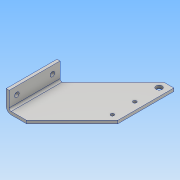
# Autodesk Inventor part: Pancake_Bracket
Saved by Autodesk Inventor 2018.1 (Build 221171000, 171)
## iProperties
Created: 2019-02-27
Part Number: Pancake_Bracket
Material: Aluminum 6061
Document SubType Name: Modeling
Designer: James
Density: 2.7 g/cm^3
Appearance: Aluminum - Flat
Author: James
Autodesk Inventor part; units mm, degrees
ref_plane "YZ Plane" through (0, 0, 0) normal (1, 0, 0) x (0, 1, 0)
ref_plane "XZ Plane" through (0, 0, 0) normal (0, 1, 0) x (-1, 0, 0)
ref_plane "XY Plane" through (0, 0, 0) normal (0, 0, 1) x (1, 0, 0)
sketch "Sketch1" plane through (0, 0, 0) normal (0, 0, 1) x (1, 0, 0)
  line L0 (0, 0) -> (65, 0)
  line L1 (65, 0) -> (65, 100)
  line L2 (65, 100) -> (0, 100)
  line L3 (0, 100) -> (0, 0)
  line L4 (0, 50) -> (5, 50)
  line L5 (5, 50) -> (55, 100)
  dimension "d0" = 65
  dimension "d1" = 100
  dimension "d28" = 45
  dimension "d29" = 50
  dimension "d30" = 5
  constraints: 12 end point, 2 horizontal, 2 parallel, 1 midpoint, 1 perpendicular, 1 point on line
  measures "d0" distance of L1.end L2.end
  measures "d1" distance of L0.end L1.end
  measures "d28" angle of L5 L2
  measures "d29" distance between parallel lines of L0 L4
  measures "d30" distance of L4.start L4.end
extrude "Extrusion1" add sketch "Sketch1" along normal blind 3 contours L3 L4 L5 L2 L1 L0
sketch "Sketch2" plane through (0, 0, 3) normal (0, 0, 1) x (1, 0, 0)
  line L0 (0, 0) -> (65, 0) projected
  line L1 (0, 0) -> (3, 0)
  line L2 (3, 0) -> (3, 50)
  line L3 (3, 50) -> (0, 50)
  line L4 (0, 50) -> (0, 0)
  dimension "d4" = 3
  dimension "d5" = 50
  constraints: 8 end point, 2 parallel, 1 horizontal, 1 perpendicular
  measures "d4" distance of L2.end L3.end
  measures "d5" distance of L1.end L2.end
extrude "Extrusion2" add sketch "Sketch2" along normal blind 17
chamfer "Chamfer2" distance 45 angle 45 1 edges at (65, 0, 1.5)
sketch "Sketch4" plane through (3, 0, 3) normal (1, 0, 0) x (0, 0, -1)
  line L0 (-17, 0) -> (-17, 50) projected
  line L1 (0, 50) -> (-17, 50) projected
  line L2 (0, 0) -> (-17, 0) projected
  point P0 (3, 0)
  point P1 (-9.5, 42.5)
  point P2 (-9.5, 7.5)
  dimension "d31" = 7.5
  dimension "d32" = 7.5
  dimension "d33" = 7.5
  dimension "d34" = 35
  constraints: 1 vertical alignment
  measures "d31" distance from line of L0 point (-9.5, 42.5)
  measures "d32" distance from line of point (-9.5, 42.5) L1
  measures "d33" distance from line of L2 point (-9.5, 7.5)
  measures "d34" distance of point (-9.5, 42.5) point (-9.5, 7.5)
hole "Hole1" at (3, 42.5, 12.5) at (3, 7.5, 12.5) direction (-1, 0, 0) diameter 4.5 end through all clearance for "Flat Head Machine Screw" size "M4" standard "Ansi Metric M Profile"
sketch "Sketch3" plane through (0, 0, 3) normal (0, 0, 1) x (1, 0, 0)
  line L0 (3, 0) -> (3, 50) projected
  line L1 (0, 50) -> (0, 0) projected
  line L2 (3, 50) -> (0, 50) projected
  point P0 (57.5, 93)
  dimension "d10" = 57.5
  dimension "d42" = 43
  measures "d10" distance from line of point (57.5, 93) L1
  measures "d42" distance from line of L2 point (57.5, 93)
hole "Hole2" at (57.5, 93, 3) direction (0, 0, -1) diameter 6 end through all
sketch "Sketch5" plane through (0, 0, 3) normal (0, 0, 1) x (1, 0, 0)
  circle A0 centre (57.5, 93) radius 3 projected
  point P0 (0, 0)
  point P1 (57.5, 69)
  point P2 (57.5, 47)
  dimension "d50" = 24
  dimension "d51" = 22
  constraints: 2 vertical alignment
  measures "d50" distance of point (57.5, 69) A0.centre
  measures "d51" distance of point (57.5, 47) point (57.5, 69)
hole "Hole3" at (57.5, 69, 3) at (57.5, 47, 3) direction (0, 0, -1) diameter 3.4 end through all clearance for "Flat Head Machine Screw" size "M3" standard "Ansi Metric M Profile"
fillet "Fillet5" radius 2 1 edges at (3, 25, 3)
fillet "Fillet6" radius 5 1 edges at (0, 25, 0)
equation "\"d33\" = d32"
body "Solid1"
